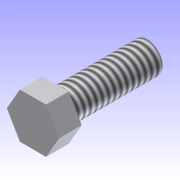
# Autodesk Inventor part: HW-00012
Saved by Autodesk Inventor 2012 (Build 160160000, 160)
## iProperties
Created: 2008-06-03
Part Number: HW-00012
Document SubType Name: Modeling
Designer: mcyr
Density: 1 g/cm^3
Description: Hex head bolt 1/4-20 x .750"
Mass: 0.962722 g
Surface Area: 6.85988 cm^2
Volume: 0.962722 cm^3
Material: Default
Title: HW-00012
Author: mcyr
Autodesk Inventor part; units mm, degrees
ref_plane "YZ Plane" through (0, 0, 0) normal (1, 0, 0) x (0, 1, 0)
ref_plane "XZ Plane" through (0, 0, 0) normal (0, 1, 0) x (-1, 0, 0)
ref_plane "XY Plane" through (0, 0, 0) normal (0, 0, 1) x (1, 0, 0)
sketch "Sketch1" plane through (0, 0, 0) normal (0, 0, 1) x (1, 0, 0)
  circle A0 centre (-0.6115, -1.5992) radius 3.175
  line L0 (-6.0374, -1.5992) -> (-3.3244, 3.0998)
  line L1 (-3.3244, 3.0998) -> (2.1015, 3.0998)
  line L2 (2.1015, 3.0998) -> (4.8145, -1.5992)
  line L3 (4.8145, -1.5992) -> (2.1015, -6.2982)
  line L4 (2.1015, -6.2982) -> (-3.3244, -6.2982)
  line L5 (-3.3244, -6.2982) -> (-6.0374, -1.5992)
  dimension "d10" = 9.398
  constraints: 12 end point, 1 centre point, 13 other
  measures "d10" distance between parallel lines of L4 L1
extrude "Extrusion1" add sketch "Sketch1" against normal blind 19.05 contours A0
extrude "Extrusion2" add sketch "Sketch1" along normal blind 4.699 contours A0 | L0 L1 L2 L3 L4 L5
thread "Thread1" size "1/4-20 UNC" class "2A" standard "ANSI Unified Screw Threads" full length
body "Solid1"
